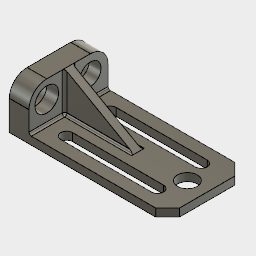
Capture History_CSA011010 (Autodesk Fusion 360 design; units mm, degrees)
Autodesk Fusion 360 part; units mm, degrees
sketch "Sketch1" plane through (0, 0, 0) normal (0, 1, 0) x (1, 0, 0) in component "Fixture"
  line L0 (100, 50) -> (-100, 50)
  line L1 (-100, 50) -> (-100, -50)
  line L2 (-100, -50) -> (100, -50)
  line L3 (100, -50) -> (100, 50)
  line L4 (100, 50) -> (-100, -50) construction
  line L5 (-100, 50) -> (100, -50) construction
  dimension "d1" = 200
  dimension "d2" = 100
  measures "d1" distance of L1.end L2.end
  measures "d2" distance of L0.end L1.end
extrude "Extrude1" add sketch "Sketch1" along normal blind 10 in component "Fixture"
sketch "Sketch2" plane through (0, 10, 0) normal (0, 1, 0) x (-1, 0, 0) in component "Fixture"
  line L0 (-100, 50) -> (-100, -50)
  line L1 (-100, -50) -> (100, -50)
  line L2 (100, -50) -> (100, 50)
  line L3 (100, 50) -> (-100, 50)
  line L4 (100, -50) -> (100, 50)
  line L5 (100, -50) -> (75, -50)
  line L6 (75, -50) -> (75, 50)
  line L7 (100, 50) -> (75, 50)
  dimension "d5" = 25
  measures "d5" distance of L1.end L5.end
extrude "Extrude2" add sketch "Sketch2" along normal blind 50 contours L1 L2 L3 L4 L5 L6 L7 in component "Fixture"
fillet "Fillet1" radius 22.5 2 edges at (-87.5, 60, 50) (-87.5, 60, -50) in component "Fixture"
sketch "Sketch3" plane through (-75, 0, 0) normal (1, 0, 0) x (0, 0, -1) in component "Fixture"
  arc A0 (50, 37.5) -> (27.5, 60) centre (27.5, 37.5) ccw
  line L0 (27.5, 60) -> (-27.5, 60)
  arc A1 (-27.5, 60) -> (-50, 37.5) centre (-27.5, 37.5) ccw
  line L1 (-50, 37.5) -> (-50, 10)
  line L2 (-50, 10) -> (50, 10)
  line L3 (50, 10) -> (50, 37.5)
  arc A2 (50, 37.5) -> (27.5, 60) centre (27.5, 37.5) ccw
  arc A3 (-27.5, 60) -> (-50, 37.5) centre (-27.5, 37.5) ccw
  circle A4 centre (-27.5, 37.5) radius 12.5
  circle A5 centre (27.5, 37.5) radius 12.5
  dimension "d9" = 25
  measures "d9" diameter of A5
extrude "Extrude3" cut sketch "Sketch3" against normal through all contours A4 | A5 in component "Fixture"
sketch "Sketch4" plane through (0, 0, 0) normal (0, 0, 1) x (1, 0, 0) in component "Fixture"
  line L0 (-75, 60) -> (-100, 60)
  line L1 (-75, 10) -> (100, 10)
  line L2 (-75, 60) -> (14.6538, 8.7692)
  line L3 (-75, 10) -> (-75, 60)
extrude "Extrude4" add sketch "Sketch4" along normal mid plane 10 in component "Fixture"
chamfer "Chamfer1" distance 15 angle 45 2 edges at (100, 5, 50) (100, 5, -50) in component "Fixture"
sketch "Sketch5" plane through (0, 10, 0) normal (0, 1, 0) x (-1, 0, 0) in component "Fixture"
  line L0 (-100, -35) -> (-85, -50)
  line L1 (-85, -50) -> (75, -50)
  line L2 (75, -50) -> (75, -5)
  line L3 (75, -5) -> (-12.5, -5)
  line L4 (-12.5, -5) -> (-12.5, 5)
  line L5 (-12.5, 5) -> (75, 5)
  line L6 (75, 5) -> (75, 50)
  line L7 (75, 50) -> (-85, 50)
  line L8 (-85, 50) -> (-100, 35)
  line L9 (-100, 35) -> (-100, -35)
  line L10 (50, 35) -> (-65, 35)
  arc A0 (-65, 35) -> (-65, 20) centre (-65, 27.5) ccw
  line L11 (-65, 20) -> (50, 20)
  arc A1 (50, 20) -> (50, 35) centre (50, 27.5) ccw
  line L12 (50, 27.5) -> (-65, 27.5) construction
  line L13 (-12.5, 0) -> (-63.9726, 0) construction
  line L14 (50, -35) -> (-65, -35)
  arc A2 (-65, -20) -> (-65, -35) centre (-65, -27.5) ccw
  line L15 (-65, -20) -> (50, -20)
  arc A3 (50, -35) -> (50, -20) centre (50, -27.5) ccw
  dimension "d14" = 15
  dimension "d15" = 22.5
  dimension "d16" = 25
  dimension "d17" = 115
  measures "d14" diameter of A0
  measures "d15" distance of L7 L12
  measures "d16" distance of L6 A1.centre
  measures "d17" distance of A1.centre A0.centre
extrude "Extrude5" cut sketch "Sketch5" against normal through all contours L10 A0 L11 A1 | L14 A2 L15 A3 in component "Fixture"
sketch "Sketch6" plane through (0, 10, 0) normal (0, 1, 0) x (-1, 0, 0) in component "Fixture"
  line L0 (-65, -20) -> (50, -20)
  arc A0 (50, -35) -> (50, -20) centre (50, -27.5) ccw
  line L1 (50, -35) -> (-65, -35)
  arc A1 (-65, -20) -> (-65, -35) centre (-65, -27.5) ccw
  line L2 (50, 20) -> (-65, 20)
  arc A2 (-65, 35) -> (-65, 20) centre (-65, 27.5) ccw
  line L3 (-65, 35) -> (50, 35)
  arc A3 (50, 20) -> (50, 35) centre (50, 27.5) ccw
  line L4 (-100, -35) -> (-85, -50)
  line L5 (-85, -50) -> (75, -50)
  line L6 (75, -50) -> (75, -5)
  line L7 (75, -5) -> (-12.5, -5)
  line L8 (-12.5, -5) -> (-12.5, 5)
  line L9 (-12.5, 5) -> (75, 5)
  line L10 (75, 5) -> (75, 50)
  line L11 (75, 50) -> (-85, 50)
  line L12 (-85, 50) -> (-100, 35)
  line L13 (-100, 35) -> (-100, -35)
  circle A4 centre (-75, 0) radius 12.5
  dimension "d19" = 25
  dimension "d20" = 75
  measures "d19" diameter of A4
  measures "d20" distance of origin A4.centre
extrude "Extrude6" cut sketch "Sketch6" against normal through all contours A4 in component "Fixture"
hole "Hole1" at (-100, 37.5, -27.5) direction (1, 0, 0) diameter 27 depth 30 tip angle 118 counterbore diameter 40 counterbore depth 10 in component "Fixture"
hole "Hole2" at (-100, 37.5, 27.5) direction (1, 0, 0) diameter 30 depth 30 tip angle 118 counterbore diameter 40 counterbore depth 10 in component "Fixture"
fillet "Fillet2" radius 3 6 edges at (-75, 10, 27.5) (-75, 35, 5) (-31.25, 10, 5) (-75, 35, -5) (-31.25, 10, -5) (-75, 10, -27.5) in component "Fixture"
component "Fixture" placed x (1, 0, 0) y (0, 1, 0) z (0, 0, 1) at (0, 0, 0)
